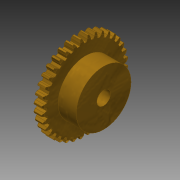
# Autodesk Inventor part: Zahnrad Messing z36
Saved by Autodesk Inventor 2017.3 (Build 213256000, 256)
## iProperties
Category: PARTsolutions
Company: MAEDLER
Created: 2018-08-20
Part Number: Zahnrad Messing z36
Material: Messing, weicher Gelbton, geschweißt
Catalog Web Link: www.cadenas.de
Description: Stzr Messing Ms58-Spur Gears, Brass, Helical Tooth Right Hand, with one-sided hub
Vendor: MAEDLER
Document SubType Name: Modeling
Designer: psadmin
Manufacturer: MAEDLER
Mass: 7.7 g
Surface Area: 8.99626 cm^2
Volume: 0.912019 cm^3
Density: 8.4428 g/cm^3
Appearance: Schweißnaht - Messing
PSOL_IDENT_0: {$CADENAS_DATA\23d-libs\maedler\antriebselemente\stirnzahnraeder\stirnzahnraeder_messing\stzr_messin
PSOL_IDENT_1: g_ms58.prj},204 {VTYP=3D},{NB=Stzr Messing Ms58 26103600},{LINA=Stzr Messing Ms58 26103600},{NN=Stzr
PSOL_IDENT_2: Messing Ms58},{DATE=03.08.2018 09:08:56},{GEOMDATE=26.07.2018 09:15:44},{VERSION=},{LINEID=390},{WB
PSOL_IDENT_3: VAR=},{WBNUMERIC=}  {NB=Stzr Messing Ms58 26103600},{LINA=Stzr Messing Ms58 26103600},{KT=DUMMY},{AR
PSOL_IDENT_4: TNR=26103600},{WST=Messing (Ms58)},{M=0.5},{Z=36},{PDF=PDF Katalogseite},{B1=2.0},{DA=19.00},{D=18.0
PSOL_IDENT_5: 0},{NL=4},{ND=12},{B=3.00},{MD=4.5},{GEW=7.700}
NN: Stzr Messing Ms58
NT: Spur Gears, Brass, Helical Tooth Right Hand, with one-sided hub
NB: Stzr Messing Ms58 26103600
NBSYN: Stzr Messing Ms58 $ARTNR.
LINA: Stzr Messing Ms58 26103600
ARTNR: 26103600
WST: Messing (Ms58)
M: 0.5
Z: 36
PDF: PDF Katalogseite
B1: 2
DA: 19
D: 18
NL: 4
ND: 12
B: 3
MD: 4.5
GEW: 7.7
SUPPLIER: MAEDLER
ARTICLENO: Stzr Messing Ms58 26103600
BOMINFO: Stzr Messing Ms58 26103600
CREATOR: CADENAS GmbH
Title: Stzr Messing Ms58 26103600
Author: Cadenas PARTsolutions
Comments: Spur Gears, Brass, Helical Tooth Right Hand, with one-sided hub
Autodesk Inventor part; units mm, degrees
ref_plane "YZ Plane" through (0, 0, 0) normal (1, 0, 0) x (0, 1, 0)
ref_plane "XZ Plane" through (0, 0, 0) normal (0, 1, 0) x (-1, 0, 0)
ref_plane "XY Plane" through (0, 0, 0) normal (0, 0, 1) x (1, 0, 0)
sketch "Skizze_1" plane through (0, 0, 0) normal (0, 0, 1) x (1, 0, 0)
  line L0 (6, 0) -> (0, 0)
  line L1 (0, 1.5) -> (6, 1.5)
  line L2 (6, 1.5) -> (6, 6)
  line L3 (6, 6) -> (2, 6)
  line L4 (2, 6) -> (2, 9)
  line L5 (2, 9) -> (1, 11.7475)
  line L6 (1, 11.7475) -> (0, 9)
  line L7 (0, 9) -> (0, 1.5)
  constraints: 16 end point
revolve "Revolution1" add sketch "Skizze_1" angle 360 about axis through (6, 0, 0) along (1, 0, 0)
sketch "Skizze_2" plane through (2, 0, 0) normal (1, 0, 0) x (0, 0, -1)
  circle A0 centre (0, 0) radius 28.5
  line L0 (-9.4769, 0.6618) -> (-8.9899, 0.4268)
  line L1 (-8.9899, 0.4268) -> (-8.4964, 0.2472)
  arc A1 (-8.4964, 0.2472) -> (-8.4964, -0.2472) centre (0, 0) ccw
  line L2 (-8.4964, -0.2472) -> (-8.9899, -0.4268)
  line L3 (-8.9899, -0.4268) -> (-9.4769, -0.6618)
  arc A2 (-9.4769, -0.6618) -> (-9.4479, -0.9939) centre (0, 0) ccw
  line L4 (-9.4479, -0.9939) -> (-8.9274, -1.1407)
  line L5 (-8.9274, -1.1407) -> (-8.4103, -1.2319)
  arc A3 (-8.4103, -1.2319) -> (-8.3244, -1.7188) centre (0, 0) ccw
  line L6 (-8.3244, -1.7188) -> (-8.7792, -1.9814)
  line L7 (-8.7792, -1.9814) -> (-9.218, -2.2974)
  arc A4 (-9.218, -2.2974) -> (-9.1317, -2.6194) centre (0, 0) ccw
  line L8 (-9.1317, -2.6194) -> (-8.5937, -2.6736)
  line L9 (-8.5937, -2.6736) -> (-8.0686, -2.6736)
  arc A5 (-8.0686, -2.6736) -> (-7.8995, -3.1383) centre (0, 0) ccw
  line L10 (-7.8995, -3.1383) -> (-8.3017, -3.4758)
  line L11 (-8.3017, -3.4758) -> (-8.679, -3.8632)
  arc A6 (-8.679, -3.8632) -> (-8.5382, -4.1653) centre (0, 0) ccw
  line L12 (-8.5382, -4.1653) -> (-7.9989, -4.1253)
  line L13 (-7.9989, -4.1253) -> (-7.4817, -4.0341)
  arc A7 (-7.4817, -4.0341) -> (-7.2345, -4.4623) centre (0, 0) ccw
  line L14 (-7.2345, -4.4623) -> (-7.572, -4.8646)
  line L15 (-7.572, -4.8646) -> (-7.8763, -5.3116)
  arc A8 (-7.8763, -5.3116) -> (-7.6852, -5.5847) centre (0, 0) ccw
  line L16 (-7.6852, -5.5847) -> (-7.161, -5.4516)
  line L17 (-7.161, -5.4516) -> (-6.6675, -5.272)
  arc A9 (-6.6675, -5.272) -> (-6.3497, -5.6508) centre (0, 0) ccw
  line L18 (-6.3497, -5.6508) -> (-6.6123, -6.1055)
  line L19 (-6.6123, -6.1055) -> (-6.8343, -6.5986)
  arc A10 (-6.8343, -6.5986) -> (-6.5986, -6.8343) centre (0, 0) ccw
  line L20 (-6.5986, -6.8343) -> (-6.1055, -6.6123)
  line L21 (-6.1055, -6.6123) -> (-5.6508, -6.3497)
  arc A11 (-5.6508, -6.3497) -> (-5.272, -6.6675) centre (0, 0) ccw
  line L22 (-5.272, -6.6675) -> (-5.4516, -7.161)
  line L23 (-5.4516, -7.161) -> (-5.5847, -7.6852)
  arc A12 (-5.5847, -7.6852) -> (-5.3116, -7.8763) centre (0, 0) ccw
  line L24 (-5.3116, -7.8763) -> (-4.8646, -7.572)
  line L25 (-4.8646, -7.572) -> (-4.4623, -7.2345)
  arc A13 (-4.4623, -7.2345) -> (-4.0341, -7.4817) centre (0, 0) ccw
  line L26 (-4.0341, -7.4817) -> (-4.1253, -7.9989)
  line L27 (-4.1253, -7.9989) -> (-4.1653, -8.5382)
  arc A14 (-4.1653, -8.5382) -> (-3.8632, -8.679) centre (0, 0) ccw
  line L28 (-3.8632, -8.679) -> (-3.4758, -8.3017)
  line L29 (-3.4758, -8.3017) -> (-3.1383, -7.8995)
  arc A15 (-3.1383, -7.8995) -> (-2.6736, -8.0686) centre (0, 0) ccw
  line L30 (-2.6736, -8.0686) -> (-2.6736, -8.5937)
  line L31 (-2.6736, -8.5937) -> (-2.6194, -9.1317)
  arc A16 (-2.6194, -9.1317) -> (-2.2974, -9.218) centre (0, 0) ccw
  line L32 (-2.2974, -9.218) -> (-1.9814, -8.7792)
  line L33 (-1.9814, -8.7792) -> (-1.7188, -8.3244)
  arc A17 (-1.7188, -8.3244) -> (-1.2319, -8.4103) centre (0, 0) ccw
  line L34 (-1.2319, -8.4103) -> (-1.1407, -8.9274)
  line L35 (-1.1407, -8.9274) -> (-0.9939, -9.4479)
  arc A18 (-0.9939, -9.4479) -> (-0.6618, -9.4769) centre (0, 0) ccw
  line L36 (-0.6618, -9.4769) -> (-0.4268, -8.9899)
  line L37 (-0.4268, -8.9899) -> (-0.2472, -8.4964)
  arc A19 (-0.2472, -8.4964) -> (0.2472, -8.4964) centre (0, 0) ccw
  line L38 (0.2472, -8.4964) -> (0.4268, -8.9899)
  line L39 (0.4268, -8.9899) -> (0.6618, -9.4769)
  arc A20 (0.6618, -9.4769) -> (0.9939, -9.4479) centre (0, 0) ccw
  line L40 (0.9939, -9.4479) -> (1.1407, -8.9274)
  line L41 (1.1407, -8.9274) -> (1.2319, -8.4103)
  arc A21 (1.2319, -8.4103) -> (1.7188, -8.3244) centre (0, 0) ccw
  line L42 (1.7188, -8.3244) -> (1.9814, -8.7792)
  line L43 (1.9814, -8.7792) -> (2.2974, -9.218)
  arc A22 (2.2974, -9.218) -> (2.6194, -9.1317) centre (0, 0) ccw
  line L44 (2.6194, -9.1317) -> (2.6736, -8.5937)
  line L45 (2.6736, -8.5937) -> (2.6736, -8.0686)
  arc A23 (2.6736, -8.0686) -> (3.1383, -7.8995) centre (0, 0) ccw
  line L46 (3.1383, -7.8995) -> (3.4758, -8.3017)
  line L47 (3.4758, -8.3017) -> (3.8632, -8.679)
  arc A24 (3.8632, -8.679) -> (4.1653, -8.5382) centre (0, 0) ccw
  line L48 (4.1653, -8.5382) -> (4.1253, -7.9989)
  line L49 (4.1253, -7.9989) -> (4.0341, -7.4817)
  arc A25 (4.0341, -7.4817) -> (4.4623, -7.2345) centre (0, 0) ccw
  line L50 (4.4623, -7.2345) -> (4.8646, -7.572)
  line L51 (4.8646, -7.572) -> (5.3116, -7.8763)
  arc A26 (5.3116, -7.8763) -> (5.5847, -7.6852) centre (0, 0) ccw
  line L52 (5.5847, -7.6852) -> (5.4516, -7.161)
  line L53 (5.4516, -7.161) -> (5.272, -6.6675)
  arc A27 (5.272, -6.6675) -> (5.6508, -6.3497) centre (0, 0) ccw
  line L54 (5.6508, -6.3497) -> (6.1055, -6.6123)
  line L55 (6.1055, -6.6123) -> (6.5986, -6.8343)
  arc A28 (6.5986, -6.8343) -> (6.8343, -6.5986) centre (0, 0) ccw
  line L56 (6.8343, -6.5986) -> (6.6123, -6.1055)
  line L57 (6.6123, -6.1055) -> (6.3497, -5.6508)
  arc A29 (6.3497, -5.6508) -> (6.6675, -5.272) centre (0, 0) ccw
  line L58 (6.6675, -5.272) -> (7.161, -5.4516)
  line L59 (7.161, -5.4516) -> (7.6852, -5.5847)
  arc A30 (7.6852, -5.5847) -> (7.8763, -5.3116) centre (0, 0) ccw
  line L60 (7.8763, -5.3116) -> (7.572, -4.8646)
  line L61 (7.572, -4.8646) -> (7.2345, -4.4623)
  arc A31 (7.2345, -4.4623) -> (7.4817, -4.0341) centre (0, 0) ccw
  line L62 (7.4817, -4.0341) -> (7.9989, -4.1253)
  line L63 (7.9989, -4.1253) -> (8.5382, -4.1653)
  arc A32 (8.5382, -4.1653) -> (8.679, -3.8632) centre (0, 0) ccw
  line L64 (8.679, -3.8632) -> (8.3017, -3.4758)
  line L65 (8.3017, -3.4758) -> (7.8995, -3.1383)
  arc A33 (7.8995, -3.1383) -> (8.0686, -2.6736) centre (0, 0) ccw
  line L66 (8.0686, -2.6736) -> (8.5937, -2.6736)
  line L67 (8.5937, -2.6736) -> (9.1317, -2.6194)
  arc A34 (9.1317, -2.6194) -> (9.218, -2.2974) centre (0, 0) ccw
  line L68 (9.218, -2.2974) -> (8.7792, -1.9814)
  line L69 (8.7792, -1.9814) -> (8.3244, -1.7188)
  arc A35 (8.3244, -1.7188) -> (8.4103, -1.2319) centre (0, 0) ccw
  line L70 (8.4103, -1.2319) -> (8.9274, -1.1407)
  line L71 (8.9274, -1.1407) -> (9.4479, -0.9939)
  arc A36 (9.4479, -0.9939) -> (9.4769, -0.6618) centre (0, 0) ccw
  line L72 (9.4769, -0.6618) -> (8.9899, -0.4268)
  line L73 (8.9899, -0.4268) -> (8.4964, -0.2472)
  arc A37 (8.4964, -0.2472) -> (8.4964, 0.2472) centre (0, 0) ccw
  line L74 (8.4964, 0.2472) -> (8.9899, 0.4268)
  line L75 (8.9899, 0.4268) -> (9.4769, 0.6618)
  arc A38 (9.4769, 0.6618) -> (9.4479, 0.9939) centre (0, 0) ccw
  line L76 (9.4479, 0.9939) -> (8.9274, 1.1407)
  line L77 (8.9274, 1.1407) -> (8.4103, 1.2319)
  arc A39 (8.4103, 1.2319) -> (8.3244, 1.7188) centre (0, 0) ccw
  line L78 (8.3244, 1.7188) -> (8.7792, 1.9814)
  line L79 (8.7792, 1.9814) -> (9.218, 2.2974)
  arc A40 (9.218, 2.2974) -> (9.1317, 2.6194) centre (0, 0) ccw
  line L80 (9.1317, 2.6194) -> (8.5937, 2.6736)
  line L81 (8.5937, 2.6736) -> (8.0686, 2.6736)
  arc A41 (8.0686, 2.6736) -> (7.8995, 3.1383) centre (0, 0) ccw
  line L82 (7.8995, 3.1383) -> (8.3017, 3.4758)
  line L83 (8.3017, 3.4758) -> (8.679, 3.8632)
  arc A42 (8.679, 3.8632) -> (8.5382, 4.1653) centre (0, 0) ccw
  line L84 (8.5382, 4.1653) -> (7.9989, 4.1253)
  line L85 (7.9989, 4.1253) -> (7.4817, 4.0341)
  arc A43 (7.4817, 4.0341) -> (7.2345, 4.4623) centre (0, 0) ccw
  line L86 (7.2345, 4.4623) -> (7.572, 4.8646)
  line L87 (7.572, 4.8646) -> (7.8763, 5.3116)
  arc A44 (7.8763, 5.3116) -> (7.6852, 5.5847) centre (0, 0) ccw
  line L88 (7.6852, 5.5847) -> (7.161, 5.4516)
  line L89 (7.161, 5.4516) -> (6.6675, 5.272)
  arc A45 (6.6675, 5.272) -> (6.3497, 5.6508) centre (0, 0) ccw
  line L90 (6.3497, 5.6508) -> (6.6123, 6.1055)
  line L91 (6.6123, 6.1055) -> (6.8343, 6.5986)
  arc A46 (6.8343, 6.5986) -> (6.5986, 6.8343) centre (0, 0) ccw
  line L92 (6.5986, 6.8343) -> (6.1055, 6.6123)
  line L93 (6.1055, 6.6123) -> (5.6508, 6.3497)
  arc A47 (5.6508, 6.3497) -> (5.272, 6.6675) centre (0, 0) ccw
  line L94 (5.272, 6.6675) -> (5.4516, 7.161)
  line L95 (5.4516, 7.161) -> (5.5847, 7.6852)
  arc A48 (5.5847, 7.6852) -> (5.3116, 7.8763) centre (0, 0) ccw
  line L96 (5.3116, 7.8763) -> (4.8646, 7.572)
  line L97 (4.8646, 7.572) -> (4.4623, 7.2345)
  arc A49 (4.4623, 7.2345) -> (4.0341, 7.4817) centre (0, 0) ccw
  line L98 (4.0341, 7.4817) -> (4.1253, 7.9989)
  line L99 (4.1253, 7.9989) -> (4.1653, 8.5382)
  arc A50 (4.1653, 8.5382) -> (3.8632, 8.679) centre (0, 0) ccw
  line L100 (3.8632, 8.679) -> (3.4758, 8.3017)
  line L101 (3.4758, 8.3017) -> (3.1383, 7.8995)
  arc A51 (3.1383, 7.8995) -> (2.6736, 8.0686) centre (0, 0) ccw
  line L102 (2.6736, 8.0686) -> (2.6736, 8.5937)
  line L103 (2.6736, 8.5937) -> (2.6194, 9.1317)
  arc A52 (2.6194, 9.1317) -> (2.2974, 9.218) centre (0, 0) ccw
  line L104 (2.2974, 9.218) -> (1.9814, 8.7792)
  line L105 (1.9814, 8.7792) -> (1.7188, 8.3244)
  arc A53 (1.7188, 8.3244) -> (1.2319, 8.4103) centre (0, 0) ccw
  line L106 (1.2319, 8.4103) -> (1.1407, 8.9274)
  line L107 (1.1407, 8.9274) -> (0.9939, 9.4479)
  arc A54 (0.9939, 9.4479) -> (0.6618, 9.4769) centre (0, 0) ccw
  line L108 (0.6618, 9.4769) -> (0.4268, 8.9899)
  line L109 (0.4268, 8.9899) -> (0.2472, 8.4964)
  arc A55 (0.2472, 8.4964) -> (-0.2472, 8.4964) centre (0, 0) ccw
  line L110 (-0.2472, 8.4964) -> (-0.4268, 8.9899)
  line L111 (-0.4268, 8.9899) -> (-0.6618, 9.4769)
  arc A56 (-0.6618, 9.4769) -> (-0.9939, 9.4479) centre (0, 0) ccw
  line L112 (-0.9939, 9.4479) -> (-1.1407, 8.9274)
  line L113 (-1.1407, 8.9274) -> (-1.2319, 8.4103)
  arc A57 (-1.2319, 8.4103) -> (-1.7188, 8.3244) centre (0, 0) ccw
  line L114 (-1.7188, 8.3244) -> (-1.9814, 8.7792)
  line L115 (-1.9814, 8.7792) -> (-2.2974, 9.218)
  arc A58 (-2.2974, 9.218) -> (-2.6194, 9.1317) centre (0, 0) ccw
  line L116 (-2.6194, 9.1317) -> (-2.6736, 8.5937)
  line L117 (-2.6736, 8.5937) -> (-2.6736, 8.0686)
  arc A59 (-2.6736, 8.0686) -> (-3.1383, 7.8995) centre (0, 0) ccw
  line L118 (-3.1383, 7.8995) -> (-3.4758, 8.3017)
  line L119 (-3.4758, 8.3017) -> (-3.8632, 8.679)
  arc A60 (-3.8632, 8.679) -> (-4.1653, 8.5382) centre (0, 0) ccw
  line L120 (-4.1653, 8.5382) -> (-4.1253, 7.9989)
  line L121 (-4.1253, 7.9989) -> (-4.0341, 7.4817)
  arc A61 (-4.0341, 7.4817) -> (-4.4623, 7.2345) centre (0, 0) ccw
  line L122 (-4.4623, 7.2345) -> (-4.8646, 7.572)
  line L123 (-4.8646, 7.572) -> (-5.3116, 7.8763)
  arc A62 (-5.3116, 7.8763) -> (-5.5847, 7.6852) centre (0, 0) ccw
  line L124 (-5.5847, 7.6852) -> (-5.4516, 7.161)
  line L125 (-5.4516, 7.161) -> (-5.272, 6.6675)
  arc A63 (-5.272, 6.6675) -> (-5.6508, 6.3497) centre (0, 0) ccw
  line L126 (-5.6508, 6.3497) -> (-6.1055, 6.6123)
  line L127 (-6.1055, 6.6123) -> (-6.5986, 6.8343)
  arc A64 (-6.5986, 6.8343) -> (-6.8343, 6.5986) centre (0, 0) ccw
  line L128 (-6.8343, 6.5986) -> (-6.6123, 6.1055)
  line L129 (-6.6123, 6.1055) -> (-6.3497, 5.6508)
  arc A65 (-6.3497, 5.6508) -> (-6.6675, 5.272) centre (0, 0) ccw
  line L130 (-6.6675, 5.272) -> (-7.161, 5.4516)
  line L131 (-7.161, 5.4516) -> (-7.6852, 5.5847)
  arc A66 (-7.6852, 5.5847) -> (-7.8763, 5.3116) centre (0, 0) ccw
  line L132 (-7.8763, 5.3116) -> (-7.572, 4.8646)
  line L133 (-7.572, 4.8646) -> (-7.2345, 4.4623)
  arc A67 (-7.2345, 4.4623) -> (-7.4817, 4.0341) centre (0, 0) ccw
  line L134 (-7.4817, 4.0341) -> (-7.9989, 4.1253)
  line L135 (-7.9989, 4.1253) -> (-8.5382, 4.1653)
  arc A68 (-8.5382, 4.1653) -> (-8.679, 3.8632) centre (0, 0) ccw
  line L136 (-8.679, 3.8632) -> (-8.3017, 3.4758)
  line L137 (-8.3017, 3.4758) -> (-7.8995, 3.1383)
  arc A69 (-7.8995, 3.1383) -> (-8.0686, 2.6736) centre (0, 0) ccw
  line L138 (-8.0686, 2.6736) -> (-8.5937, 2.6736)
  line L139 (-8.5937, 2.6736) -> (-9.1317, 2.6194)
  arc A70 (-9.1317, 2.6194) -> (-9.218, 2.2974) centre (0, 0) ccw
  line L140 (-9.218, 2.2974) -> (-8.7792, 1.9814)
  line L141 (-8.7792, 1.9814) -> (-8.3244, 1.7188)
  arc A71 (-8.3244, 1.7188) -> (-8.4103, 1.2319) centre (0, 0) ccw
  line L142 (-8.4103, 1.2319) -> (-8.9274, 1.1407)
  line L143 (-8.9274, 1.1407) -> (-9.4479, 0.9939)
  arc A72 (-9.4479, 0.9939) -> (-9.4769, 0.6618) centre (0, 0) ccw
  constraints: 288 end point, 144 point on circle, 73 centre point
extrude "Extrusion1" cut sketch "Skizze_2" along normal mid plane 12
body "Solid1"
